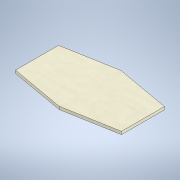
# Autodesk Inventor part: Speaker
Saved by Autodesk Inventor 2021 (Build 250183000, 183)
## iProperties
Created: 2023-03-16
Part Number: Speaker
Material: Paper
Document SubType Name: Modeling
Designer: Bradley
Density: 0.93 g/cm^3
Appearance: Cardboard - Chipboard
Author: Bradley
Autodesk Inventor part; units mm, degrees
ref_plane "YZ Plane" through (0, 0, 0) normal (1, 0, 0) x (0, 1, 0)
ref_plane "XZ Plane" through (0, 0, 0) normal (0, 1, 0) x (-1, 0, 0)
ref_plane "XY Plane" through (0, 0, 0) normal (0, 0, 1) x (1, 0, 0)
sketch "Sketch1" plane through (0, 0, 0) normal (0, 1, 0) x (-1, 0, 0)
  line L0 (30.85, -12.5) -> (30.85, 12.5)
  line L1 (30.85, 12.5) -> (0, 18)
  line L2 (0, 18) -> (-30.85, 12.5)
  line L3 (-30.85, 12.5) -> (-30.85, -12.5)
  line L4 (-30.85, -12.5) -> (0, -18)
  line L5 (0, -18) -> (30.85, -12.5)
  point P0 (0, 0)
  point P1 (30.85, 0)
  point P2 (-30.85, 0)
  dimension "d0" = 61.7
  dimension "d1" = 25
  dimension "d2" = 36
  constraints: 12 end point, 3 equal length, 2 horizontal alignment, 2 midpoint, 2 parallel, 1 vertical, 1 vertical alignment
  measures "d0" distance between parallel lines of L3 L0
  measures "d1" distance of L2.end L3.end
  measures "d2" distance of L1.end L4.end
extrude "Extrusion1" add sketch "Sketch1" along normal mid plane 1.7
body "Solid1"
